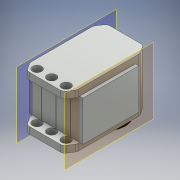
# Autodesk Inventor part: servo
Saved by Autodesk Inventor 2016 (Build 200138000, 138)
## iProperties
Created: 2016-05-17
Part Number: servo
Material: Generic
Document SubType Name: Modeling
Designer: Hamid Osooli
Density: 1 g/cm^3
Appearance: Default
Mass: 17.7811 g
Surface Area: 45.9491 cm^2
Volume: 17.7811 cm^3
Author: Hamid Osooli
Autodesk Inventor part; units mm, degrees
ref_plane "YZ Plane" through (0, 0, 0) normal (1, 0, 0) x (0, 1, 0)
ref_plane "XZ Plane" through (0, 0, 0) normal (0, 1, 0) x (-1, 0, 0)
sketch "Sketch2" plane through (0, 0, 0) normal (0, 0, 1) x (1, 0, 0)
  line L0 (5.0984, -40.3499) -> (19.0293, -40.3499)
  line L1 (22.6152, -35.9079) -> (22.6152, -8.9424)
  line L2 (18.9317, -4.3499) -> (5.0984, -4.3499)
  line L3 (1.5125, -8.792) -> (1.5125, -35.9079)
  line L4 (3.421, -5.2607) -> (1.8351, -7.7028)
  line L5 (3.421, -39.4392) -> (1.8351, -36.9971)
  line L6 (20.7066, -39.4392) -> (22.2925, -36.9971)
  line L7 (22.2925, -7.8531) -> (20.609, -5.2607)
  arc A0 (5.0984, -4.3499) -> (3.421, -5.2607) centre (5.0984, -6.3499) ccw
  arc A1 (1.8351, -7.7028) -> (1.5125, -8.792) centre (3.5125, -8.792) ccw
  arc A2 (20.609, -5.2607) -> (18.9317, -4.3499) centre (18.9317, -6.3499) ccw
  arc A3 (22.6152, -8.9424) -> (22.2925, -7.8531) centre (20.6152, -8.9424) ccw
  arc A4 (1.5125, -35.9079) -> (1.8351, -36.9971) centre (3.5125, -35.9079) ccw
  arc A5 (3.421, -39.4392) -> (5.0984, -40.3499) centre (5.0984, -38.3499) ccw
  arc A6 (19.0293, -40.3499) -> (20.7066, -39.4392) centre (19.0293, -38.3499) ccw
  arc A7 (22.2925, -36.9971) -> (22.6152, -35.9079) centre (20.6152, -35.9079) ccw
  point P0 (0, 0)
  point P1 (22.6152, -4.3499)
  point P2 (22.6152, -40.3499)
  dimension "d116" = 36
  dimension "d117" = 2
  dimension "d119" = 2
  constraints: 16 end point, 16 point on circle, 16 tangent, 8 centre point, 6 equal radius, 4 point on line, 2 parallel, 1 horizontal, 1 perpendicular
  measures "d116" distance of point (22.615, -4.35) point (22.615, -40.35)
  measures "d117" radius of A0
  measures "d119" radius of A4
extrude "Extrusion1" add sketch "Sketch2" along normal blind 24
sketch "Sketch3" plane through (0, 0, 0) normal (0, 0, 1) x (1, 0, 0)
  circle A0 centre (12.015, -12.869) radius 8.5
  point P0 (0, 0)
  dimension "d244" = 17
  constraints: 1 centre point
  measures "d244" diameter of A0
extrude "Extrusion2" add sketch "Sketch3" against normal blind 3
sketch "Sketch6" plane through (0, 0, 0) normal (1, 0, 0) x (0, 1, 0)
  line L0 (-40.3499, 0) -> (-40.3499, 24) projected
  line L1 (-40.3499, 3) -> (-35.3499, 3)
  line L2 (-35.3499, 3) -> (-35.3499, 21)
  line L3 (-35.3499, 21) -> (-40.3499, 21)
  line L4 (-40.3499, 21) -> (-40.3499, 3)
  point P0 (0, 0)
  dimension "d221" = 5
  dimension "d222" = 18
  constraints: 8 end point, 2 parallel, 1 horizontal, 1 perpendicular, 1 point on line
  measures "d221" distance of L3.end L2.end
  measures "d222" distance of L2.end L1.end
extrude "Extrusion3" cut sketch "Sketch6" along normal up to next
ref_plane "Work Plane2" through (1.5125, -8.792, 24) normal (-1, 0, 0) x (0, -1, 0)
sketch "Sketch8" plane through (1.5125, -8.792, 24) normal (-1, 0, 0) x (0, -1, 0)
  line L0 (26.5579, -3) -> (26.5579, -21) projected
  line L1 (26.5579, -3) -> (1.5579, -3)
  line L2 (1.5579, -3) -> (1.5579, -21)
  line L3 (1.5579, -21) -> (26.5579, -21)
  line L4 (26.5579, -21) -> (26.5579, -3)
  dimension "d243" = 25
  constraints: 8 end point, 2 parallel, 1 horizontal, 1 perpendicular
  measures "d243" distance of L3.end L2.end
extrude "Extrusion4" add sketch "Sketch8" along normal blind 1.4485
ref_plane "Work Plane3" through (22.6152, -35.9079, 24) normal (1, 0, 0) x (0, 1, 0)
sketch "Sketch9" plane through (22.6152, -35.9079, 24) normal (1, 0, 0) x (0, 1, 0)
  line L0 (0.5579, -21) -> (25.5579, -21)
  line L1 (25.5579, -21) -> (25.5579, -3)
  line L2 (25.5579, -3) -> (0.5579, -3)
  line L3 (0.5579, -3) -> (0.5579, -21)
  dimension "d239" = 25
  dimension "d240" = 18
  constraints: 8 end point, 2 parallel, 1 horizontal, 1 perpendicular
  measures "d239" distance of L2.end L1.end
  measures "d240" distance of L1.end L0.end
extrude "Extrusion5" add sketch "Sketch9" along normal blind 1.4485
sketch "Sketch10" plane through (0, 0, 0) normal (0, 0, 1) x (1, 0, 0)
  circle A0 centre (12.0638, -37.347) radius 2
  circle A1 centre (5.564, -37.347) radius 2
  circle A2 centre (18.564, -37.347) radius 2
  point P0 (0, 0)
  dimension "d245" = 4
  dimension "d246" = 4
  dimension "d247" = 4
  constraints: 3 centre point
  measures "d245" diameter of A0
  measures "d246" diameter of A1
  measures "d247" diameter of A2
extrude "Extrusion7" cut sketch "Sketch10" along normal blind 24
body "Solid1"
